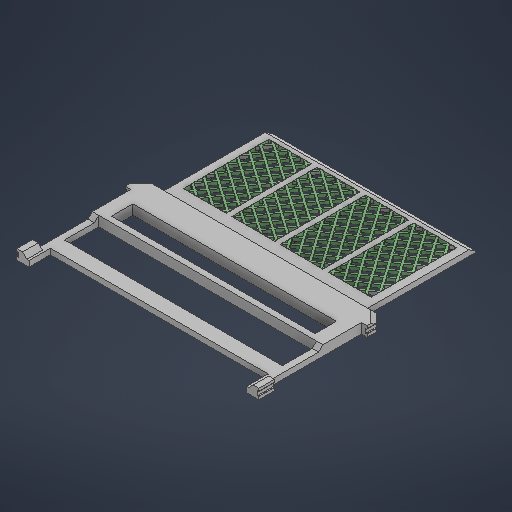
# Autodesk Inventor part: SACMI PH1500 FILLER BOX GRID-DRIVING
Saved by Autodesk Inventor 2025 (Build 290162000, 162)
## iProperties
Created: 2024-05-03
Part Number: SACMI PH1500 FILLER BOX GRID-DRIVING
Material: Generic
Document SubType Name: Modeling
Designer: zulet
Density: 1 g/cm^3
Appearance: Smooth - Medium Gray
Author: zulet
Autodesk Inventor part; units mm, degrees
(part 1 of 2)
ref_plane "YZ Plane" through (0, 0, 0) normal (1, 0, 0) x (0, 1, 0)
ref_plane "XZ Plane" through (0, 0, 0) normal (0, 1, 0) x (-1, 0, 0)
ref_plane "XY Plane" through (0, 0, 0) normal (0, 0, 1) x (1, 0, 0)
sketch "Sketch1" plane through (0, 0, 0) normal (0, 1, 0) x (-1, 0, 0)
  line L0 (-2029.8955, 1380.0763) -> (2005.9504, 1380.0763) construction
  line L1 (2005.9504, 1380.0763) -> (2005.9504, -2689.5627) construction
  line L2 (2005.9504, -2689.5627) -> (-2029.8955, -2689.5627) construction
  line L3 (-2029.8955, -2689.5627) -> (-2029.8955, 1380.0763) construction
  line L4 (810, 0) -> (765, 0)
  line L5 (715, -900) -> (780, -900)
  line L6 (780, -900) -> (850, -830)
  line L7 (850, -830) -> (850, -760)
  line L8 (850, -760) -> (810, -760)
  line L9 (810, -760) -> (810, 0)
  line L10 (715, -900) -> (715, -1610)
  line L11 (715, -1610) -> (0, -1610)
  line L12 (0, -1610) -> (0, -680)
  line L13 (0, -680) -> (715, -680)
  line L14 (765, -490) -> (0, -490)
  line L15 (0, -490) -> (0, -530)
  line L16 (0, -530) -> (715, -530)
  line L17 (715, -530) -> (715, -680)
  line L18 (765, -490) -> (765, -250)
  line L19 (765, -250) -> (0, -250)
  line L20 (0, -250) -> (0, -150)
  line L21 (0, -150) -> (765, -150)
  line L22 (765, -150) -> (765, 0)
  line L23 (810, 0) -> (850, 0)
  line L24 (850, 0) -> (850, -110)
  line L25 (850, -110) -> (810, -110)
  line L26 (810, -110) -> (810, 0)
  line L27 (0, 0) -> (0, -1610) construction
  line L28 (0, 0) -> (850, 0) construction
  line L29 (715, -900) -> (715, -680)
  line L30 (765, -490) -> (810, -490)
  line L31 (715, -900) -> (0, -900)
  point P0 (830, -110)
  point P1 (715, -605)
  point P2 (810, -110)
  point P3 (0, -900)
  dimension "d1" = 4035.8459
  dimension "d24" = 45
  dimension "d25" = 150
  dimension "d26" = 100
  dimension "d27" = 240
  dimension "d28" = 40
  dimension "d29" = 150
  dimension "d32" = 810
  dimension "d33" = 110
  dimension "d43" = 650
  dimension "d45" = 140
  dimension "d46" = 45
  dimension "d48" = 70
  dimension "d49" = 40
  dimension "d50" = 95
  dimension "d57" = 780
  constraints: 56 end point, 13 perpendicular, 7 horizontal, 6 collinear, 4 point on line, 3 vertical, 2 midpoint, 2 parallel, 2 other
  measures "d1" distance of L1.end L2.end
  measures "d24" distance between parallel lines of L22 L9
  measures "d25" distance between parallel lines of L4 L21
  measures "d26" distance between parallel lines of L19 L21
  measures "d27" distance between parallel lines of L14 L19
  measures "d28" distance between parallel lines of L16 L14
  measures "d29" distance between parallel lines of L13 L16
  measures "d32" distance between parallel lines of L27 L9
  measures "d33" distance of L23.end L24.end
  measures "d43" distance from line of point (830, -110) L8
  measures "d45" distance between parallel lines of L8 L5
  measures "d46" angle of L5 L6
  measures "d48" distance of L6.end L7.end
  measures "d49" distance between parallel lines of L9 L24
  measures "d50" distance from line of L9 point (715, -605)
  measures "d57" distance from line of L11 L6.end
extrude "Extrusion1" add sketch "Sketch1" along normal blind 70 contours L23 L24 L25 L9 | L9 L8 L7 L6 L5 L29 L17 L16 L15 L14 L30 | L31 L12 L13 L29
extrude "Extrusion3" add sketch "Sketch1" along normal blind 40 contours L9 L30 L18 L19 L20 L21 L22 L4 | L31 L12 L13 L29 | L10 L11 L12 L31
sketch "Sketch2" plane through (0, 40, 0) normal (0, 1, 0) x (1, 0, 0)
  line L0 (-660, 1580) -> (-360, 1580)
  line L1 (-360, 1580) -> (-360, 980)
  line L2 (-360, 980) -> (-660, 980)
  line L3 (-660, 980) -> (-660, 1580)
  line L4 (0, 1610) -> (-715, 1610) projected
  line L5 (-850, 830) -> (-850, 760) projected
  line L6 (-320, 980) -> (-20, 980)
  line L7 (-20, 980) -> (-20, 1580)
  line L8 (-20, 1580) -> (-320, 1580)
  line L9 (-320, 1580) -> (-320, 980)
  point P0 (0, 0)
  dimension "d58" = 300
  dimension "d59" = 600
  dimension "d60" = 30
  dimension "d61" = 190
  dimension "d62" = 300
  dimension "d63" = 600
  dimension "d64" = 40
  dimension "d65" = 30
  constraints: 16 end point, 4 parallel, 2 horizontal, 2 perpendicular
  measures "d58" distance of L1.end L2.end
  measures "d59" distance of L0.end L1.end
  measures "d60" distance between parallel lines of L4 L0
  measures "d61" distance between parallel lines of L3 L5
  measures "d62" distance of L8.end L7.end
  measures "d63" distance of L7.end L6.end
  measures "d64" distance between parallel lines of L1 L9
  measures "d65" distance between parallel lines of L4 L8
extrude "Extrusion4" cut sketch "Sketch2" against normal blind 40
sketch "Sketch3" plane through (0, 40, 0) normal (0, 1, 0) x (1, 0, 0)
  line L0 (317.5928, 1321.2787) -> (276.6352, 1349.9575)
  line L1 (276.6352, 1349.9575) -> (305.314, 1390.9151)
  line L2 (305.314, 1390.9151) -> (346.2716, 1362.2363)
  line L3 (346.2716, 1362.2363) -> (317.5928, 1321.2787)
  line L4 (-360, 980) -> (-660, 980) projected
  line L5 (264.3479, 1358.5611) -> (223.3903, 1387.24)
  line L6 (223.3903, 1387.24) -> (252.0691, 1428.1976)
  line L7 (252.0691, 1428.1976) -> (293.0267, 1399.5187)
  line L8 (293.0267, 1399.5187) -> (264.3479, 1358.5611)
  line L9 (211.103, 1395.8436) -> (170.1454, 1424.5224)
  line L10 (170.1454, 1424.5224) -> (198.8242, 1465.48)
  line L11 (198.8242, 1465.48) -> (239.7818, 1436.8012)
  line L12 (239.7818, 1436.8012) -> (211.103, 1395.8436)
  line L13 (157.8581, 1433.1261) -> (116.9005, 1461.8049)
  line L14 (116.9005, 1461.8049) -> (145.5794, 1502.7625)
  line L15 (145.5794, 1502.7625) -> (186.537, 1474.0837)
  line L16 (186.537, 1474.0837) -> (157.8581, 1433.1261)
  line L17 (104.6133, 1470.4085) -> (63.6557, 1499.0874)
  line L18 (63.6557, 1499.0874) -> (92.3345, 1540.045)
  line L19 (92.3345, 1540.045) -> (133.2921, 1511.3661)
  line L20 (133.2921, 1511.3661) -> (104.6133, 1470.4085)
  line L21 (51.3684, 1507.691) -> (10.4108, 1536.3698)
  line L22 (10.4108, 1536.3698) -> (39.0896, 1577.3274)
  line L23 (39.0896, 1577.3274) -> (80.0472, 1548.6486)
  line L24 (80.0472, 1548.6486) -> (51.3684, 1507.691)
  line L25 (-1.8765, 1544.9735) -> (-42.8341, 1573.6523)
  line L26 (-42.8341, 1573.6523) -> (-14.1553, 1614.6099)
  line L27 (-14.1553, 1614.6099) -> (26.8023, 1585.9311)
  line L28 (26.8023, 1585.9311) -> (-1.8765, 1544.9735)
  line L29 (-55.1214, 1582.2559) -> (-96.079, 1610.9348)
  line L30 (-96.079, 1610.9348) -> (-67.4002, 1651.8924)
  line L31 (-67.4002, 1651.8924) -> (-26.4426, 1623.2135)
  line L32 (-26.4426, 1623.2135) -> (-55.1214, 1582.2559)
  line L33 (-108.3663, 1619.5384) -> (-149.3239, 1648.2172)
  line L34 (-149.3239, 1648.2172) -> (-120.6451, 1689.1748)
  line L35 (-120.6451, 1689.1748) -> (-79.6874, 1660.496)
  line L36 (-79.6874, 1660.496) -> (-108.3663, 1619.5384)
  line L37 (-161.6112, 1656.8209) -> (-202.5688, 1685.4997)
  line L38 (-202.5688, 1685.4997) -> (-173.8899, 1726.4573)
  line L39 (-173.8899, 1726.4573) -> (-132.9323, 1697.7785)
  line L40 (-132.9323, 1697.7785) -> (-161.6112, 1656.8209)
  line L41 (-214.856, 1694.1033) -> (-255.8136, 1722.7822)
  line L42 (-255.8136, 1722.7822) -> (-227.1348, 1763.7398)
  line L43 (-227.1348, 1763.7398) -> (-186.1772, 1735.0609)
  line L44 (-186.1772, 1735.0609) -> (-214.856, 1694.1033)
  line L45 (-268.1009, 1731.3858) -> (-309.0585, 1760.0646)
  line L46 (-309.0585, 1760.0646) -> (-280.3797, 1801.0222)
  line L47 (-280.3797, 1801.0222) -> (-239.4221, 1772.3434)
  line L48 (-239.4221, 1772.3434) -> (-268.1009, 1731.3858)
  line L49 (-321.3458, 1768.6683) -> (-362.3034, 1797.3471)
  line L50 (-362.3034, 1797.3471) -> (-333.6246, 1838.3047)
  line L51 (-333.6246, 1838.3047) -> (-292.667, 1809.6259)
  line L52 (-292.667, 1809.6259) -> (-321.3458, 1768.6683)
  line L53 (-374.5907, 1805.9508) -> (-415.5483, 1834.6296)
  line L54 (-415.5483, 1834.6296) -> (-386.8695, 1875.5872)
  line L55 (-386.8695, 1875.5872) -> (-345.9119, 1846.9084)
  line L56 (-345.9119, 1846.9084) -> (-374.5907, 1805.9508)
  line L57 (-427.8356, 1843.2332) -> (-468.7932, 1871.912)
  line L58 (-468.7932, 1871.912) -> (-440.1143, 1912.8696)
  line L59 (-440.1143, 1912.8696) -> (-399.1567, 1884.1908)
  line L60 (-399.1567, 1884.1908) -> (-427.8356, 1843.2332)
  line L61 (280.3103, 1268.0338) -> (239.3527, 1296.7126)
  line L62 (239.3527, 1296.7126) -> (268.0315, 1337.6702)
  line L63 (268.0315, 1337.6702) -> (308.9891, 1308.9914)
  line L64 (308.9891, 1308.9914) -> (280.3103, 1268.0338)
  line L65 (227.0654, 1305.3162) -> (186.1078, 1333.9951)
  line L66 (186.1078, 1333.9951) -> (214.7867, 1374.9527)
  line L67 (214.7867, 1374.9527) -> (255.7443, 1346.2739)
  line L68 (255.7443, 1346.2739) -> (227.0654, 1305.3162)
  line L69 (173.8206, 1342.5987) -> (132.863, 1371.2775)
  line L70 (132.863, 1371.2775) -> (161.5418, 1412.2351)
  line L71 (161.5418, 1412.2351) -> (202.4994, 1383.5563)
  line L72 (202.4994, 1383.5563) -> (173.8206, 1342.5987)
  line L73 (120.5757, 1379.8812) -> (79.6181, 1408.56)
  line L74 (79.6181, 1408.56) -> (108.2969, 1449.5176)
  line L75 (108.2969, 1449.5176) -> (149.2545, 1420.8388)
  line L76 (149.2545, 1420.8388) -> (120.5757, 1379.8812)
  line L77 (67.3308, 1417.1637) -> (26.3732, 1445.8425)
  line L78 (26.3732, 1445.8425) -> (55.052, 1486.8001)
  line L79 (55.052, 1486.8001) -> (96.0096, 1458.1213)
  line L80 (96.0096, 1458.1213) -> (67.3308, 1417.1637)
  line L81 (14.0859, 1454.4461) -> (-26.8717, 1483.1249)
  line L82 (-26.8717, 1483.1249) -> (1.8071, 1524.0825)
  line L83 (1.8071, 1524.0825) -> (42.7647, 1495.4037)
  line L84 (42.7647, 1495.4037) -> (14.0859, 1454.4461)
  line L85 (-39.159, 1491.7286) -> (-80.1166, 1520.4074)
  line L86 (-80.1166, 1520.4074) -> (-51.4378, 1561.365)
  line L87 (-51.4378, 1561.365) -> (-10.4802, 1532.6862)
  line L88 (-10.4802, 1532.6862) -> (-39.159, 1491.7286)
  line L89 (-92.4039, 1529.0111) -> (-133.3615, 1557.6899)
  line L90 (-133.3615, 1557.6899) -> (-104.6826, 1598.6475)
  line L91 (-104.6826, 1598.6475) -> (-63.725, 1569.9687)
  line L92 (-63.725, 1569.9687) -> (-92.4039, 1529.0111)
  line L93 (-145.6487, 1566.2935) -> (-186.6063, 1594.9723)
  line L94 (-186.6063, 1594.9723) -> (-157.9275, 1635.93)
  line L95 (-157.9275, 1635.93) -> (-116.9699, 1607.2511)
  line L96 (-116.9699, 1607.2511) -> (-145.6487, 1566.2935)
  line L97 (-198.8936, 1603.576) -> (-239.8512, 1632.2548)
  line L98 (-239.8512, 1632.2548) -> (-211.1724, 1673.2124)
  line L99 (-211.1724, 1673.2124) -> (-170.2148, 1644.5336)
  line L100 (-170.2148, 1644.5336) -> (-198.8936, 1603.576)
  line L101 (-252.1385, 1640.8585) -> (-293.0961, 1669.5373)
  line L102 (-293.0961, 1669.5373) -> (-264.4173, 1710.4949)
  line L103 (-264.4173, 1710.4949) -> (-223.4597, 1681.8161)
  line L104 (-223.4597, 1681.8161) -> (-252.1385, 1640.8585)
  line L105 (-305.3834, 1678.1409) -> (-346.341, 1706.8198)
  line L106 (-346.341, 1706.8198) -> (-317.6622, 1747.7774)
  line L107 (-317.6622, 1747.7774) -> (-276.7046, 1719.0985)
  line L108 (-276.7046, 1719.0985) -> (-305.3834, 1678.1409)
  line L109 (-358.6283, 1715.4234) -> (-399.5859, 1744.1022)
  line L110 (-399.5859, 1744.1022) -> (-370.9071, 1785.0598)
  line L111 (-370.9071, 1785.0598) -> (-329.9494, 1756.381)
  line L112 (-329.9494, 1756.381) -> (-358.6283, 1715.4234)
  line L113 (-411.8732, 1752.7059) -> (-452.8308, 1781.3847)
  line L114 (-452.8308, 1781.3847) -> (-424.1519, 1822.3423)
  line L115 (-424.1519, 1822.3423) -> (-383.1943, 1793.6635)
  line L116 (-383.1943, 1793.6635) -> (-411.8732, 1752.7059)
  line L117 (-465.118, 1789.9883) -> (-506.0756, 1818.6672)
  line L118 (-506.0756, 1818.6672) -> (-477.3968, 1859.6248)
  line L119 (-477.3968, 1859.6248) -> (-436.4392, 1830.9459)
  line L120 (-436.4392, 1830.9459) -> (-465.118, 1789.9883)
  line L121 (243.0279, 1214.7889) -> (202.0703, 1243.4677)
  line L122 (202.0703, 1243.4677) -> (230.7491, 1284.4253)
  line L123 (230.7491, 1284.4253) -> (271.7067, 1255.7465)
  line L124 (271.7067, 1255.7465) -> (243.0279, 1214.7889)
  line L125 (189.783, 1252.0714) -> (148.8254, 1280.7502)
  line L126 (148.8254, 1280.7502) -> (177.5042, 1321.7078)
  line L127 (177.5042, 1321.7078) -> (218.4618, 1293.029)
  line L128 (218.4618, 1293.029) -> (189.783, 1252.0714)
  line L129 (136.5381, 1289.3538) -> (95.5805, 1318.0327)
  line L130 (95.5805, 1318.0327) -> (124.2593, 1358.9903)
  line L131 (124.2593, 1358.9903) -> (165.2169, 1330.3114)
  line L132 (165.2169, 1330.3114) -> (136.5381, 1289.3538)
  line L133 (83.2932, 1326.6363) -> (42.3356, 1355.3151)
  line L134 (42.3356, 1355.3151) -> (71.0144, 1396.2727)
  line L135 (71.0144, 1396.2727) -> (111.972, 1367.5939)
  line L136 (111.972, 1367.5939) -> (83.2932, 1326.6363)
  line L137 (30.0483, 1363.9188) -> (-10.9093, 1392.5976)
  line L138 (-10.9093, 1392.5976) -> (17.7695, 1433.5552)
  line L139 (17.7695, 1433.5552) -> (58.7271, 1404.8764)
  line L140 (58.7271, 1404.8764) -> (30.0483, 1363.9188)
  line L141 (-23.1966, 1401.2012) -> (-64.1542, 1429.8801)
  line L142 (-64.1542, 1429.8801) -> (-35.4753, 1470.8377)
  line L143 (-35.4753, 1470.8377) -> (5.4823, 1442.1588)
  line L144 (5.4823, 1442.1588) -> (-23.1966, 1401.2012)
  line L145 (-76.4414, 1438.4837) -> (-117.399, 1467.1625)
  line L146 (-117.399, 1467.1625) -> (-88.7202, 1508.1201)
  line L147 (-88.7202, 1508.1201) -> (-47.7626, 1479.4413)
  line L148 (-47.7626, 1479.4413) -> (-76.4414, 1438.4837)
  line L149 (-129.6863, 1475.7662) -> (-170.6439, 1504.445)
  line L150 (-170.6439, 1504.445) -> (-141.9651, 1545.4026)
  line L151 (-141.9651, 1545.4026) -> (-101.0075, 1516.7238)
  line L152 (-101.0075, 1516.7238) -> (-129.6863, 1475.7662)
  line L153 (-182.9312, 1513.0486) -> (-223.8888, 1541.7275)
  line L154 (-223.8888, 1541.7275) -> (-195.21, 1582.6851)
  line L155 (-195.21, 1582.6851) -> (-154.2524, 1554.0062)
  line L156 (-154.2524, 1554.0062) -> (-182.9312, 1513.0486)
  line L157 (-236.1761, 1550.3311) -> (-277.1337, 1579.0099)
  line L158 (-277.1337, 1579.0099) -> (-248.4549, 1619.9675)
  line L159 (-248.4549, 1619.9675) -> (-207.4973, 1591.2887)
  line L160 (-207.4973, 1591.2887) -> (-236.1761, 1550.3311)
  line L161 (-289.421, 1587.6136) -> (-330.3786, 1616.2924)
  line L162 (-330.3786, 1616.2924) -> (-301.6998, 1657.25)
  line L163 (-301.6998, 1657.25) -> (-260.7422, 1628.5712)
  line L164 (-260.7422, 1628.5712) -> (-289.421, 1587.6136)
  line L165 (-342.6659, 1624.896) -> (-383.6235, 1653.5749)
  line L166 (-383.6235, 1653.5749) -> (-354.9446, 1694.5325)
  line L167 (-354.9446, 1694.5325) -> (-313.987, 1665.8537)
  line L168 (-313.987, 1665.8537) -> (-342.6659, 1624.896)
  line L169 (-395.9107, 1662.1785) -> (-436.8683, 1690.8573)
  line L170 (-436.8683, 1690.8573) -> (-408.1895, 1731.8149)
  line L171 (-408.1895, 1731.8149) -> (-367.2319, 1703.1361)
  line L172 (-367.2319, 1703.1361) -> (-395.9107, 1662.1785)
  line L173 (-449.1556, 1699.461) -> (-490.1132, 1728.1398)
  line L174 (-490.1132, 1728.1398) -> (-461.4344, 1769.0974)
  line L175 (-461.4344, 1769.0974) -> (-420.4768, 1740.4186)
  line L176 (-420.4768, 1740.4186) -> (-449.1556, 1699.461)
  line L177 (-502.4005, 1736.7435) -> (-543.3581, 1765.4223)
  line L178 (-543.3581, 1765.4223) -> (-514.6793, 1806.3799)
  line L179 (-514.6793, 1806.3799) -> (-473.7217, 1777.7011)
  line L180 (-473.7217, 1777.7011) -> (-502.4005, 1736.7435)
  line L181 (205.7454, 1161.544) -> (164.7878, 1190.2228)
  line L182 (164.7878, 1190.2228) -> (193.4666, 1231.1804)
  line L183 (193.4666, 1231.1804) -> (234.4242, 1202.5016)
  line L184 (234.4242, 1202.5016) -> (205.7454, 1161.544)
  line L185 (152.5005, 1198.8265) -> (111.5429, 1227.5053)
  line L186 (111.5429, 1227.5053) -> (140.2217, 1268.4629)
  line L187 (140.2217, 1268.4629) -> (181.1793, 1239.7841)
  line L188 (181.1793, 1239.7841) -> (152.5005, 1198.8265)
  line L189 (99.2556, 1236.109) -> (58.298, 1264.7878)
  line L190 (58.298, 1264.7878) -> (86.9768, 1305.7454)
  line L191 (86.9768, 1305.7454) -> (127.9344, 1277.0666)
  line L192 (127.9344, 1277.0666) -> (99.2556, 1236.109)
  line L193 (46.0107, 1273.3914) -> (5.0531, 1302.0702)
  line L194 (5.0531, 1302.0702) -> (33.732, 1343.0278)
  line L195 (33.732, 1343.0278) -> (74.6896, 1314.349)
  line L196 (74.6896, 1314.349) -> (46.0107, 1273.3914)
  line L197 (-7.2341, 1310.6739) -> (-48.1917, 1339.3527)
  line L198 (-48.1917, 1339.3527) -> (-19.5129, 1380.3103)
  line L199 (-19.5129, 1380.3103) -> (21.4447, 1351.6315)
  line L200 (21.4447, 1351.6315) -> (-7.2341, 1310.6739)
  line L201 (-60.479, 1347.9564) -> (-101.4366, 1376.6352)
  line L202 (-101.4366, 1376.6352) -> (-72.7578, 1417.5928)
  line L203 (-72.7578, 1417.5928) -> (-31.8002, 1388.914)
  line L204 (-31.8002, 1388.914) -> (-60.479, 1347.9564)
  line L205 (-113.7239, 1385.2388) -> (-154.6815, 1413.9176)
  line L206 (-154.6815, 1413.9176) -> (-126.0027, 1454.8752)
  line L207 (-126.0027, 1454.8752) -> (-85.0451, 1426.1964)
  line L208 (-85.0451, 1426.1964) -> (-113.7239, 1385.2388)
  line L209 (-166.9688, 1422.5213) -> (-207.9264, 1451.2001)
  line L210 (-207.9264, 1451.2001) -> (-179.2476, 1492.1577)
  line L211 (-179.2476, 1492.1577) -> (-138.29, 1463.4789)
  line L212 (-138.29, 1463.4789) -> (-166.9688, 1422.5213)
  line L213 (-220.2137, 1459.8038) -> (-261.1713, 1488.4826)
  line L214 (-261.1713, 1488.4826) -> (-232.4925, 1529.4402)
  line L215 (-232.4925, 1529.4402) -> (-191.5349, 1500.7614)
  line L216 (-191.5349, 1500.7614) -> (-220.2137, 1459.8038)
  line L217 (-273.4586, 1497.0862) -> (-314.4162, 1525.7651)
  line L218 (-314.4162, 1525.7651) -> (-285.7373, 1566.7227)
  line L219 (-285.7373, 1566.7227) -> (-244.7797, 1538.0438)
  line L220 (-244.7797, 1538.0438) -> (-273.4586, 1497.0862)
  line L221 (-326.7034, 1534.3687) -> (-367.661, 1563.0475)
  line L222 (-367.661, 1563.0475) -> (-338.9822, 1604.0051)
  line L223 (-338.9822, 1604.0051) -> (-298.0246, 1575.3263)
  line L224 (-298.0246, 1575.3263) -> (-326.7034, 1534.3687)
  line L225 (-379.9483, 1571.6512) -> (-420.9059, 1600.33)
  line L226 (-420.9059, 1600.33) -> (-392.2271, 1641.2876)
  line L227 (-392.2271, 1641.2876) -> (-351.2695, 1612.6088)
  line L228 (-351.2695, 1612.6088) -> (-379.9483, 1571.6512)
  line L229 (-433.1932, 1608.9336) -> (-474.1508, 1637.6125)
  line L230 (-474.1508, 1637.6125) -> (-445.472, 1678.5701)
  line L231 (-445.472, 1678.5701) -> (-404.5144, 1649.8912)
  line L232 (-404.5144, 1649.8912) -> (-433.1932, 1608.9336)
  line L233 (-486.4381, 1646.2161) -> (-527.3957, 1674.8949)
  line L234 (-527.3957, 1674.8949) -> (-498.7169, 1715.8525)
  line L235 (-498.7169, 1715.8525) -> (-457.7593, 1687.1737)
  line L236 (-457.7593, 1687.1737) -> (-486.4381, 1646.2161)
  line L237 (-539.683, 1683.4986) -> (-580.6406, 1712.1774)
  line L238 (-580.6406, 1712.1774) -> (-551.9618, 1753.135)
  line L239 (-551.9618, 1753.135) -> (-511.0042, 1724.4562)
  line L240 (-511.0042, 1724.4562) -> (-539.683, 1683.4986)
  line L241 (168.4629, 1108.2991) -> (127.5053, 1136.978)
  line L242 (127.5053, 1136.978) -> (156.1841, 1177.9356)
  line L243 (156.1841, 1177.9356) -> (197.1417, 1149.2567)
  line L244 (197.1417, 1149.2567) -> (168.4629, 1108.2991)
  line L245 (115.218, 1145.5816) -> (74.2604, 1174.2604)
  line L246 (74.2604, 1174.2604) -> (102.9393, 1215.218)
  line L247 (102.9393, 1215.218) -> (143.8969, 1186.5392)
  line L248 (143.8969, 1186.5392) -> (115.218, 1145.5816)
  line L249 (61.9732, 1182.8641) -> (21.0156, 1211.5429)
  line L250 (21.0156, 1211.5429) -> (49.6944, 1252.5005)
  line L251 (49.6944, 1252.5005) -> (90.652, 1223.8217)
  line L252 (90.652, 1223.8217) -> (61.9732, 1182.8641)
  line L253 (8.7283, 1220.1465) -> (-32.2293, 1248.8254)
  line L254 (-32.2293, 1248.8254) -> (-3.5505, 1289.783)
  line L255 (-3.5505, 1289.783) -> (37.4071, 1261.1041)
  line L256 (37.4071, 1261.1041) -> (8.7283, 1220.1465)
  line L257 (-44.5166, 1257.429) -> (-85.4742, 1286.1078)
  line L258 (-85.4742, 1286.1078) -> (-56.7954, 1327.0654)
  line L259 (-56.7954, 1327.0654) -> (-15.8378, 1298.3866)
  line L260 (-15.8378, 1298.3866) -> (-44.5166, 1257.429)
  line L261 (-97.7615, 1294.7115) -> (-138.7191, 1323.3903)
  line L262 (-138.7191, 1323.3903) -> (-110.0403, 1364.3479)
  line L263 (-110.0403, 1364.3479) -> (-69.0827, 1335.6691)
  line L264 (-69.0827, 1335.6691) -> (-97.7615, 1294.7115)
  line L265 (-151.0064, 1331.9939) -> (-191.964, 1360.6728)
  line L266 (-191.964, 1360.6728) -> (-163.2852, 1401.6304)
  line L267 (-163.2852, 1401.6304) -> (-122.3276, 1372.9515)
  line L268 (-122.3276, 1372.9515) -> (-151.0064, 1331.9939)
  line L269 (-204.2513, 1369.2764) -> (-245.2089, 1397.9552)
  line L270 (-245.2089, 1397.9552) -> (-216.53, 1438.9128)
  line L271 (-216.53, 1438.9128) -> (-175.5724, 1410.234)
  line L272 (-175.5724, 1410.234) -> (-204.2513, 1369.2764)
  line L273 (-257.4961, 1406.5589) -> (-298.4537, 1435.2377)
  line L274 (-298.4537, 1435.2377) -> (-269.7749, 1476.1953)
  line L275 (-269.7749, 1476.1953) -> (-228.8173, 1447.5165)
  line L276 (-228.8173, 1447.5165) -> (-257.4961, 1406.5589)
  line L277 (-310.741, 1443.8413) -> (-351.6986, 1472.5202)
  line L278 (-351.6986, 1472.5202) -> (-323.0198, 1513.4778)
  line L279 (-323.0198, 1513.4778) -> (-282.0622, 1484.7989)
  line L280 (-282.0622, 1484.7989) -> (-310.741, 1443.8413)
  line L281 (-363.9859, 1481.1238) -> (-404.9435, 1509.8026)
  line L282 (-404.9435, 1509.8026) -> (-376.2647, 1550.7602)
  line L283 (-376.2647, 1550.7602) -> (-335.3071, 1522.0814)
  line L284 (-335.3071, 1522.0814) -> (-363.9859, 1481.1238)
  line L285 (-417.2308, 1518.4063) -> (-458.1884, 1547.0851)
  line L286 (-458.1884, 1547.0851) -> (-429.5096, 1588.0427)
  line L287 (-429.5096, 1588.0427) -> (-388.552, 1559.3639)
  line L288 (-388.552, 1559.3639) -> (-417.2308, 1518.4063)
  line L289 (-470.4757, 1555.6888) -> (-511.4333, 1584.3676)
  line L290 (-511.4333, 1584.3676) -> (-482.7545, 1625.3252)
  line L291 (-482.7545, 1625.3252) -> (-441.7969, 1596.6464)
  line L292 (-441.7969, 1596.6464) -> (-470.4757, 1555.6888)
  line L293 (-523.7206, 1592.9712) -> (-564.6782, 1621.65)
  line L294 (-564.6782, 1621.65) -> (-535.9993, 1662.6076)
  line L295 (-535.9993, 1662.6076) -> (-495.0417, 1633.9288)
  line L296 (-495.0417, 1633.9288) -> (-523.7206, 1592.9712)
  line L297 (-576.9654, 1630.2537) -> (-617.923, 1658.9325)
  line L298 (-617.923, 1658.9325) -> (-589.2442, 1699.8901)
  line L299 (-589.2442, 1699.8901) -> (-548.2866, 1671.2113)
  line L300 (-548.2866, 1671.2113) -> (-576.9654, 1630.2537)
  line L301 (131.1805, 1055.0542) -> (90.2228, 1083.7331)
  line L302 (90.2228, 1083.7331) -> (118.9017, 1124.6907)
  line L303 (118.9017, 1124.6907) -> (159.8593, 1096.0119)
  line L304 (159.8593, 1096.0119) -> (131.1805, 1055.0542)
  line L305 (77.9356, 1092.3367) -> (36.978, 1121.0155)
  line L306 (36.978, 1121.0155) -> (65.6568, 1161.9731)
  line L307 (65.6568, 1161.9731) -> (106.6144, 1133.2943)
  line L308 (106.6144, 1133.2943) -> (77.9356, 1092.3367)
  line L309 (24.6907, 1129.6192) -> (-16.2669, 1158.298)
  line L310 (-16.2669, 1158.298) -> (12.4119, 1199.2556)
  line L311 (12.4119, 1199.2556) -> (53.3695, 1170.5768)
  line L312 (53.3695, 1170.5768) -> (24.6907, 1129.6192)
  line L313 (-28.5542, 1166.9017) -> (-69.5118, 1195.5805)
  line L314 (-69.5118, 1195.5805) -> (-40.833, 1236.5381)
  line L315 (-40.833, 1236.5381) -> (0.1246, 1207.8593)
  line L316 (0.1246, 1207.8593) -> (-28.5542, 1166.9017)
  line L317 (-81.7991, 1204.1841) -> (-122.7567, 1232.8629)
  line L318 (-122.7567, 1232.8629) -> (-94.0779, 1273.8205)
  line L319 (-94.0779, 1273.8205) -> (-53.1203, 1245.1417)
  line L320 (-53.1203, 1245.1417) -> (-81.7991, 1204.1841)
  line L321 (-135.044, 1241.4666) -> (-176.0016, 1270.1454)
  line L322 (-176.0016, 1270.1454) -> (-147.3227, 1311.103)
  line L323 (-147.3227, 1311.103) -> (-106.3651, 1282.4242)
  line L324 (-106.3651, 1282.4242) -> (-135.044, 1241.4666)
  line L325 (-188.2888, 1278.7491) -> (-229.2464, 1307.4279)
  line L326 (-229.2464, 1307.4279) -> (-200.5676, 1348.3855)
  line L327 (-200.5676, 1348.3855) -> (-159.61, 1319.7067)
  line L328 (-159.61, 1319.7067) -> (-188.2888, 1278.7491)
  line L329 (-241.5337, 1316.0315) -> (-282.4913, 1344.7103)
  line L330 (-282.4913, 1344.7103) -> (-253.8125, 1385.668)
  line L331 (-253.8125, 1385.668) -> (-212.8549, 1356.9891)
  line L332 (-212.8549, 1356.9891) -> (-241.5337, 1316.0315)
  line L333 (-294.7786, 1353.314) -> (-335.7362, 1381.9928)
  line L334 (-335.7362, 1381.9928) -> (-307.0574, 1422.9504)
  line L335 (-307.0574, 1422.9504) -> (-266.0998, 1394.2716)
  line L336 (-266.0998, 1394.2716) -> (-294.7786, 1353.314)
  line L337 (-348.0235, 1390.5965) -> (-388.9811, 1419.2753)
  line L338 (-388.9811, 1419.2753) -> (-360.3023, 1460.2329)
  line L339 (-360.3023, 1460.2329) -> (-319.3447, 1431.5541)
  line L340 (-319.3447, 1431.5541) -> (-348.0235, 1390.5965)
  line L341 (-401.2684, 1427.8789) -> (-442.226, 1456.5578)
  line L342 (-442.226, 1456.5578) -> (-413.5472, 1497.5154)
  line L343 (-413.5472, 1497.5154) -> (-372.5896, 1468.8365)
  line L344 (-372.5896, 1468.8365) -> (-401.2684, 1427.8789)
  line L345 (-454.5133, 1465.1614) -> (-495.4709, 1493.8402)
  line L346 (-495.4709, 1493.8402) -> (-466.792, 1534.7978)
  line L347 (-466.792, 1534.7978) -> (-425.8344, 1506.119)
  line L348 (-425.8344, 1506.119) -> (-454.5133, 1465.1614)
  line L349 (-507.7581, 1502.4439) -> (-548.7157, 1531.1227)
  line L350 (-548.7157, 1531.1227) -> (-520.0369, 1572.0803)
  line L351 (-520.0369, 1572.0803) -> (-479.0793, 1543.4015)
  line L352 (-479.0793, 1543.4015) -> (-507.7581, 1502.4439)
  line L353 (-561.003, 1539.7263) -> (-601.9606, 1568.4052)
  line L354 (-601.9606, 1568.4052) -> (-573.2818, 1609.3628)
  line L355 (-573.2818, 1609.3628) -> (-532.3242, 1580.6839)
  line L356 (-532.3242, 1580.6839) -> (-561.003, 1539.7263)
  line L357 (-614.2479, 1577.0088) -> (-655.2055, 1605.6876)
  line L358 (-655.2055, 1605.6876) -> (-626.5267, 1646.6452)
  line L359 (-626.5267, 1646.6452) -> (-585.5691, 1617.9664)
  line L360 (-585.5691, 1617.9664) -> (-614.2479, 1577.0088)
  line L361 (93.898, 1001.8094) -> (52.9404, 1030.4882)
  line L362 (52.9404, 1030.4882) -> (81.6192, 1071.4458)
  line L363 (81.6192, 1071.4458) -> (122.5768, 1042.767)
  line L364 (122.5768, 1042.767) -> (93.898, 1001.8094)
  line L365 (40.6531, 1039.0918) -> (-0.3045, 1067.7707)
  line L366 (-0.3045, 1067.7707) -> (28.3743, 1108.7283)
  line L367 (28.3743, 1108.7283) -> (69.3319, 1080.0494)
  line L368 (69.3319, 1080.0494) -> (40.6531, 1039.0918)
  line L369 (-12.5918, 1076.3743) -> (-53.5494, 1105.0531)
  line L370 (-53.5494, 1105.0531) -> (-24.8706, 1146.0107)
  line L371 (-24.8706, 1146.0107) -> (16.087, 1117.3319)
  line L372 (16.087, 1117.3319) -> (-12.5918, 1076.3743)
  line L373 (-65.8367, 1113.6568) -> (-106.7943, 1142.3356)
  line L374 (-106.7943, 1142.3356) -> (-78.1154, 1183.2932)
  line L375 (-78.1154, 1183.2932) -> (-37.1578, 1154.6144)
  line L376 (-37.1578, 1154.6144) -> (-65.8367, 1113.6568)
  line L377 (-119.0815, 1150.9392) -> (-160.0392, 1179.6181)
  line L378 (-160.0392, 1179.6181) -> (-131.3603, 1220.5757)
  line L379 (-131.3603, 1220.5757) -> (-90.4027, 1191.8968)
  line L380 (-90.4027, 1191.8968) -> (-119.0815, 1150.9392)
  line L381 (-172.3264, 1188.2217) -> (-213.284, 1216.9005)
  line L382 (-213.284, 1216.9005) -> (-184.6052, 1257.8581)
  line L383 (-184.6052, 1257.8581) -> (-143.6476, 1229.1793)
  line L384 (-143.6476, 1229.1793) -> (-172.3264, 1188.2217)
  line L385 (-225.5713, 1225.5042) -> (-266.5289, 1254.183)
  line L386 (-266.5289, 1254.183) -> (-237.8501, 1295.1406)
  line L387 (-237.8501, 1295.1406) -> (-196.8925, 1266.4618)
  line L388 (-196.8925, 1266.4618) -> (-225.5713, 1225.5042)
  line L389 (-278.8162, 1262.7866) -> (-319.7738, 1291.4655)
  line L390 (-319.7738, 1291.4655) -> (-291.095, 1332.4231)
  line L391 (-291.095, 1332.4231) -> (-250.1374, 1303.7442)
  line L392 (-250.1374, 1303.7442) -> (-278.8162, 1262.7866)
  line L393 (-332.0611, 1300.0691) -> (-373.0187, 1328.7479)
  line L394 (-373.0187, 1328.7479) -> (-344.3399, 1369.7055)
  line L395 (-344.3399, 1369.7055) -> (-303.3823, 1341.0267)
  line L396 (-303.3823, 1341.0267) -> (-332.0611, 1300.0691)
  line L397 (-385.306, 1337.3516) -> (-426.2636, 1366.0304)
  line L398 (-426.2636, 1366.0304) -> (-397.5847, 1406.988)
  line L399 (-397.5847, 1406.988) -> (-356.6271, 1378.3092)
  line L400 (-356.6271, 1378.3092) -> (-385.306, 1337.3516)
  line L401 (-438.5508, 1374.6341) -> (-479.5084, 1403.3129)
  line L402 (-479.5084, 1403.3129) -> (-450.8296, 1444.2705)
  line L403 (-450.8296, 1444.2705) -> (-409.872, 1415.5917)
  line L404 (-409.872, 1415.5917) -> (-438.5508, 1374.6341)
  line L405 (-491.7957, 1411.9165) -> (-532.7533, 1440.5953)
  line L406 (-532.7533, 1440.5953) -> (-504.0745, 1481.5529)
  line L407 (-504.0745, 1481.5529) -> (-463.1169, 1452.8741)
  line L408 (-463.1169, 1452.8741) -> (-491.7957, 1411.9165)
  line L409 (-545.0406, 1449.199) -> (-585.9982, 1477.8778)
  line L410 (-585.9982, 1477.8778) -> (-557.3194, 1518.8354)
  line L411 (-557.3194, 1518.8354) -> (-516.3618, 1490.1566)
  line L412 (-516.3618, 1490.1566) -> (-545.0406, 1449.199)
  line L413 (-598.2855, 1486.4815) -> (-639.2431, 1515.1603)
  line L414 (-639.2431, 1515.1603) -> (-610.5643, 1556.1179)
  line L415 (-610.5643, 1556.1179) -> (-569.6067, 1527.4391)
  line L416 (-569.6067, 1527.4391) -> (-598.2855, 1486.4815)
  line L417 (-651.5304, 1523.7639) -> (-692.488, 1552.4427)
  line L418 (-692.488, 1552.4427) -> (-663.8092, 1593.4003)
  line L419 (-663.8092, 1593.4003) -> (-622.8516, 1564.7215)
  line L420 (-622.8516, 1564.7215) -> (-651.5304, 1523.7639)
  line L421 (56.6155, 948.5645) -> (15.6579, 977.2433)
  line L422 (15.6579, 977.2433) -> (44.3367, 1018.2009)
  line L423 (44.3367, 1018.2009) -> (85.2943, 989.5221)
  line L424 (85.2943, 989.5221) -> (56.6155, 948.5645)
  line L425 (3.3706, 985.847) -> (-37.587, 1014.5258)
  line L426 (-37.587, 1014.5258) -> (-8.9081, 1055.4834)
  line L427 (-8.9081, 1055.4834) -> (32.0495, 1026.8046)
  line L428 (32.0495, 1026.8046) -> (3.3706, 985.847)
  line L429 (-49.8743, 1023.1294) -> (-90.8319, 1051.8082)
  line L430 (-90.8319, 1051.8082) -> (-62.153, 1092.7658)
  line L431 (-62.153, 1092.7658) -> (-21.1954, 1064.087)
  line L432 (-21.1954, 1064.087) -> (-49.8743, 1023.1294)
  line L433 (-103.1191, 1060.4119) -> (-144.0767, 1089.0907)
  line L434 (-144.0767, 1089.0907) -> (-115.3979, 1130.0483)
  line L435 (-115.3979, 1130.0483) -> (-74.4403, 1101.3695)
  line L436 (-74.4403, 1101.3695) -> (-103.1191, 1060.4119)
  line L437 (-156.364, 1097.6944) -> (-197.3216, 1126.3732)
  line L438 (-197.3216, 1126.3732) -> (-168.6428, 1167.3308)
  line L439 (-168.6428, 1167.3308) -> (-127.6852, 1138.652)
  line L440 (-127.6852, 1138.652) -> (-156.364, 1097.6944)
  line L441 (-209.6089, 1134.9768) -> (-250.5665, 1163.6556)
  line L442 (-250.5665, 1163.6556) -> (-221.8877, 1204.6132)
  line L443 (-221.8877, 1204.6132) -> (-180.9301, 1175.9344)
  line L444 (-180.9301, 1175.9344) -> (-209.6089, 1134.9768)
  line L445 (-262.8538, 1172.2593) -> (-303.8114, 1200.9381)
  line L446 (-303.8114, 1200.9381) -> (-275.1326, 1241.8957)
  line L447 (-275.1326, 1241.8957) -> (-234.175, 1213.2169)
  line L448 (-234.175, 1213.2169) -> (-262.8538, 1172.2593)
  line L449 (-316.0987, 1209.5418) -> (-357.0563, 1238.2206)
  line L450 (-357.0563, 1238.2206) -> (-328.3774, 1279.1782)
  line L451 (-328.3774, 1279.1782) -> (-287.4198, 1250.4994)
  line L452 (-287.4198, 1250.4994) -> (-316.0987, 1209.5418)
  line L453 (-369.3435, 1246.8242) -> (-410.3012, 1275.5031)
  line L454 (-410.3012, 1275.5031) -> (-381.6223, 1316.4607)
  line L455 (-381.6223, 1316.4607) -> (-340.6647, 1287.7818)
  line L456 (-340.6647, 1287.7818) -> (-369.3435, 1246.8242)
  line L457 (-422.5884, 1284.1067) -> (-463.546, 1312.7855)
  line L458 (-463.546, 1312.7855) -> (-434.8672, 1353.7431)
  line L459 (-434.8672, 1353.7431) -> (-393.9096, 1325.0643)
  line L460 (-393.9096, 1325.0643) -> (-422.5884, 1284.1067)
  line L461 (-475.8333, 1321.3892) -> (-516.7909, 1350.068)
  line L462 (-516.7909, 1350.068) -> (-488.1121, 1391.0256)
  line L463 (-488.1121, 1391.0256) -> (-447.1545, 1362.3468)
  line L464 (-447.1545, 1362.3468) -> (-475.8333, 1321.3892)
  line L465 (-529.0782, 1358.6716) -> (-570.0358, 1387.3505)
  line L466 (-570.0358, 1387.3505) -> (-541.357, 1428.3081)
  line L467 (-541.357, 1428.3081) -> (-500.3994, 1399.6292)
  line L468 (-500.3994, 1399.6292) -> (-529.0782, 1358.6716)
  line L469 (-582.3231, 1395.9541) -> (-623.2807, 1424.6329)
  line L470 (-623.2807, 1424.6329) -> (-594.6019, 1465.5905)
  line L471 (-594.6019, 1465.5905) -> (-553.6443, 1436.9117)
  line L472 (-553.6443, 1436.9117) -> (-582.3231, 1395.9541)
  line L473 (-635.568, 1433.2366) -> (-676.5256, 1461.9154)
  line L474 (-676.5256, 1461.9154) -> (-647.8467, 1502.873)
  line L475 (-647.8467, 1502.873) -> (-606.8891, 1474.1942)
  line L476 (-606.8891, 1474.1942) -> (-635.568, 1433.2366)
  line L477 (-688.8128, 1470.519) -> (-729.7704, 1499.1979)
  line L478 (-729.7704, 1499.1979) -> (-701.0916, 1540.1555)
  line L479 (-701.0916, 1540.1555) -> (-660.134, 1511.4766)
  line L480 (-660.134, 1511.4766) -> (-688.8128, 1470.519)
  line L481 (19.333, 895.3196) -> (-21.6246, 923.9984)
  line L482 (-21.6246, 923.9984) -> (7.0543, 964.956)
  line L483 (7.0543, 964.956) -> (48.0119, 936.2772)
  line L484 (48.0119, 936.2772) -> (19.333, 895.3196)
  line L485 (-33.9118, 932.6021) -> (-74.8694, 961.2809)
  line L486 (-74.8694, 961.2809) -> (-46.1906, 1002.2385)
  line L487 (-46.1906, 1002.2385) -> (-5.233, 973.5597)
  line L488 (-5.233, 973.5597) -> (-33.9118, 932.6021)
  line L489 (-87.1567, 969.8845) -> (-128.1143, 998.5634)
  line L490 (-128.1143, 998.5634) -> (-99.4355, 1039.521)
  line L491 (-99.4355, 1039.521) -> (-58.4779, 1010.8421)
  line L492 (-58.4779, 1010.8421) -> (-87.1567, 969.8845)
  line L493 (-140.4016, 1007.167) -> (-181.3592, 1035.8458)
  line L494 (-181.3592, 1035.8458) -> (-152.6804, 1076.8034)
  line L495 (-152.6804, 1076.8034) -> (-111.7228, 1048.1246)
  line L496 (-111.7228, 1048.1246) -> (-140.4016, 1007.167)
  line L497 (-193.6465, 1044.4495) -> (-234.6041, 1073.1283)
  line L498 (-234.6041, 1073.1283) -> (-205.9253, 1114.0859)
  line L499 (-205.9253, 1114.0859) -> (-164.9677, 1085.4071)
  line L500 (-164.9677, 1085.4071) -> (-193.6465, 1044.4495)
  line L501 (-246.8914, 1081.7319) -> (-287.849, 1110.4108)
  line L502 (-287.849, 1110.4108) -> (-259.1701, 1151.3684)
  line L503 (-259.1701, 1151.3684) -> (-218.2125, 1122.6895)
  line L504 (-218.2125, 1122.6895) -> (-246.8914, 1081.7319)
  line L505 (-300.1363, 1119.0144) -> (-341.0939, 1147.6932)
  line L506 (-341.0939, 1147.6932) -> (-312.415, 1188.6508)
  line L507 (-312.415, 1188.6508) -> (-271.4574, 1159.972)
  line L508 (-271.4574, 1159.972) -> (-300.1363, 1119.0144)
  line L509 (-353.3811, 1156.2969) -> (-394.3387, 1184.9757)
  line L510 (-394.3387, 1184.9757) -> (-365.6599, 1225.9333)
  line L511 (-365.6599, 1225.9333) -> (-324.7023, 1197.2545)
  line L512 (-324.7023, 1197.2545) -> (-353.3811, 1156.2969)
  line L513 (-406.626, 1193.5793) -> (-447.5836, 1222.2582)
  line L514 (-447.5836, 1222.2582) -> (-418.9048, 1263.2158)
  line L515 (-418.9048, 1263.2158) -> (-377.9472, 1234.5369)
  line L516 (-377.9472, 1234.5369) -> (-406.626, 1193.5793)
  line L517 (-459.8709, 1230.8618) -> (-500.8285, 1259.5406)
  line L518 (-500.8285, 1259.5406) -> (-472.1497, 1300.4982)
  line L519 (-472.1497, 1300.4982) -> (-431.1921, 1271.8194)
  line L520 (-431.1921, 1271.8194) -> (-459.8709, 1230.8618)
  line L521 (-513.1158, 1268.1443) -> (-554.0734, 1296.8231)
  line L522 (-554.0734, 1296.8231) -> (-525.3946, 1337.7807)
  line L523 (-525.3946, 1337.7807) -> (-484.437, 1309.1019)
  line L524 (-484.437, 1309.1019) -> (-513.1158, 1268.1443)
  line L525 (-566.3607, 1305.4268) -> (-607.3183, 1334.1056)
  line L526 (-607.3183, 1334.1056) -> (-578.6394, 1375.0632)
  line L527 (-578.6394, 1375.0632) -> (-537.6818, 1346.3844)
  line L528 (-537.6818, 1346.3844) -> (-566.3607, 1305.4268)
  line L529 (-619.6055, 1342.7092) -> (-660.5632, 1371.388)
  line L530 (-660.5632, 1371.388) -> (-631.8843, 1412.3456)
  line L531 (-631.8843, 1412.3456) -> (-590.9267, 1383.6668)
  line L532 (-590.9267, 1383.6668) -> (-619.6055, 1342.7092)
  line L533 (-672.8504, 1379.9917) -> (-713.808, 1408.6705)
  line L534 (-713.808, 1408.6705) -> (-685.1292, 1449.6281)
  line L535 (-685.1292, 1449.6281) -> (-644.1716, 1420.9493)
  line L536 (-644.1716, 1420.9493) -> (-672.8504, 1379.9917)
  line L537 (-726.0953, 1417.2742) -> (-767.0529, 1445.953)
  line L538 (-767.0529, 1445.953) -> (-738.3741, 1486.9106)
  line L539 (-738.3741, 1486.9106) -> (-697.4165, 1458.2318)
  line L540 (-697.4165, 1458.2318) -> (-726.0953, 1417.2742)
  line L541 (-17.9494, 842.0747) -> (-58.907, 870.7535)
  line L542 (-58.907, 870.7535) -> (-30.2282, 911.7111)
  line L543 (-30.2282, 911.7111) -> (10.7294, 883.0323)
  line L544 (10.7294, 883.0323) -> (-17.9494, 842.0747)
  line L545 (-71.1943, 879.3572) -> (-112.1519, 908.036)
  line L546 (-112.1519, 908.036) -> (-83.4731, 948.9936)
  line L547 (-83.4731, 948.9936) -> (-42.5155, 920.3148)
  line L548 (-42.5155, 920.3148) -> (-71.1943, 879.3572)
  line L549 (-124.4392, 916.6397) -> (-165.3968, 945.3185)
  line L550 (-165.3968, 945.3185) -> (-136.718, 986.2761)
  line L551 (-136.718, 986.2761) -> (-95.7604, 957.5973)
  line L552 (-95.7604, 957.5973) -> (-124.4392, 916.6397)
  line L553 (-177.6841, 953.9221) -> (-218.6417, 982.6009)
  line L554 (-218.6417, 982.6009) -> (-189.9629, 1023.5585)
  line L555 (-189.9629, 1023.5585) -> (-149.0052, 994.8797)
  line L556 (-149.0052, 994.8797) -> (-177.6841, 953.9221)
  line L557 (-230.929, 991.2046) -> (-271.8866, 1019.8834)
  line L558 (-271.8866, 1019.8834) -> (-243.2077, 1060.841)
  line L559 (-243.2077, 1060.841) -> (-202.2501, 1032.1622)
  line L560 (-202.2501, 1032.1622) -> (-230.929, 991.2046)
  line L561 (-284.1738, 1028.4871) -> (-325.1314, 1057.1659)
  line L562 (-325.1314, 1057.1659) -> (-296.4526, 1098.1235)
  line L563 (-296.4526, 1098.1235) -> (-255.495, 1069.4447)
  line L564 (-255.495, 1069.4447) -> (-284.1738, 1028.4871)
  line L565 (-337.4187, 1065.7695) -> (-378.3763, 1094.4483)
  line L566 (-378.3763, 1094.4483) -> (-349.6975, 1135.406)
  line L567 (-349.6975, 1135.406) -> (-308.7399, 1106.7271)
  line L568 (-308.7399, 1106.7271) -> (-337.4187, 1065.7695)
  line L569 (-390.6636, 1103.052) -> (-431.6212, 1131.7308)
  line L570 (-431.6212, 1131.7308) -> (-402.9424, 1172.6884)
  line L571 (-402.9424, 1172.6884) -> (-361.9848, 1144.0096)
  line L572 (-361.9848, 1144.0096) -> (-390.6636, 1103.052)
  line L573 (-443.9085, 1140.3345) -> (-484.8661, 1169.0133)
  line L574 (-484.8661, 1169.0133) -> (-456.1873, 1209.9709)
  line L575 (-456.1873, 1209.9709) -> (-415.2297, 1181.2921)
  line L576 (-415.2297, 1181.2921) -> (-443.9085, 1140.3345)
  line L577 (-497.1534, 1177.6169) -> (-538.111, 1206.2958)
  line L578 (-538.111, 1206.2958) -> (-509.4321, 1247.2534)
  line L579 (-509.4321, 1247.2534) -> (-468.4745, 1218.5745)
  line L580 (-468.4745, 1218.5745) -> (-497.1534, 1177.6169)
  line L581 (-550.3983, 1214.8994) -> (-591.3559, 1243.5782)
  line L582 (-591.3559, 1243.5782) -> (-562.677, 1284.5358)
  line L583 (-562.677, 1284.5358) -> (-521.7194, 1255.857)
  line L584 (-521.7194, 1255.857) -> (-550.3983, 1214.8994)
  line L585 (-603.6431, 1252.1819) -> (-644.6007, 1280.8607)
  line L586 (-644.6007, 1280.8607) -> (-615.9219, 1321.8183)
  line L587 (-615.9219, 1321.8183) -> (-574.9643, 1293.1395)
  line L588 (-574.9643, 1293.1395) -> (-603.6431, 1252.1819)
  line L589 (-656.888, 1289.4643) -> (-697.8456, 1318.1432)
  line L590 (-697.8456, 1318.1432) -> (-669.1668, 1359.1008)
  line L591 (-669.1668, 1359.1008) -> (-628.2092, 1330.4219)
  line L592 (-628.2092, 1330.4219) -> (-656.888, 1289.4643)
  line L593 (-710.1329, 1326.7468) -> (-751.0905, 1355.4256)
  line L594 (-751.0905, 1355.4256) -> (-722.4117, 1396.3832)
  line L595 (-722.4117, 1396.3832) -> (-681.4541, 1367.7044)
  line L596 (-681.4541, 1367.7044) -> (-710.1329, 1326.7468)
  line L597 (-763.3778, 1364.0293) -> (-804.3354, 1392.7081)
  line L598 (-804.3354, 1392.7081) -> (-775.6566, 1433.6657)
  line L599 (-775.6566, 1433.6657) -> (-734.699, 1404.9869)
  line L600 (-734.699, 1404.9869) -> (-763.3778, 1364.0293)
  line L601 (-55.2319, 788.8298) -> (-96.1895, 817.5087)
  line L602 (-96.1895, 817.5087) -> (-67.5107, 858.4663)
  line L603 (-67.5107, 858.4663) -> (-26.5531, 829.7874)
  line L604 (-26.5531, 829.7874) -> (-55.2319, 788.8298)
  line L605 (-108.4768, 826.1123) -> (-149.4344, 854.7911)
  line L606 (-149.4344, 854.7911) -> (-120.7556, 895.7487)
  line L607 (-120.7556, 895.7487) -> (-79.798, 867.0699)
  line L608 (-79.798, 867.0699) -> (-108.4768, 826.1123)
  line L609 (-161.7217, 863.3948) -> (-202.6793, 892.0736)
  line L610 (-202.6793, 892.0736) -> (-174.0004, 933.0312)
  line L611 (-174.0004, 933.0312) -> (-133.0428, 904.3524)
  line L612 (-133.0428, 904.3524) -> (-161.7217, 863.3948)
  line L613 (-214.9665, 900.6772) -> (-255.9241, 929.3561)
  line L614 (-255.9241, 929.3561) -> (-227.2453, 970.3137)
  line L615 (-227.2453, 970.3137) -> (-186.2877, 941.6348)
  line L616 (-186.2877, 941.6348) -> (-214.9665, 900.6772)
  line L617 (-268.2114, 937.9597) -> (-309.169, 966.6385)
  line L618 (-309.169, 966.6385) -> (-280.4902, 1007.5961)
  line L619 (-280.4902, 1007.5961) -> (-239.5326, 978.9173)
  line L620 (-239.5326, 978.9173) -> (-268.2114, 937.9597)
  line L621 (-321.4563, 975.2422) -> (-362.4139, 1003.921)
  line L622 (-362.4139, 1003.921) -> (-333.7351, 1044.8786)
  line L623 (-333.7351, 1044.8786) -> (-292.7775, 1016.1998)
  line L624 (-292.7775, 1016.1998) -> (-321.4563, 975.2422)
  line L625 (-374.7012, 1012.5246) -> (-415.6588, 1041.2035)
  line L626 (-415.6588, 1041.2035) -> (-386.98, 1082.1611)
  line L627 (-386.98, 1082.1611) -> (-346.0224, 1053.4822)
  line L628 (-346.0224, 1053.4822) -> (-374.7012, 1012.5246)
  line L629 (-427.9461, 1049.8071) -> (-468.9037, 1078.4859)
  line L630 (-468.9037, 1078.4859) -> (-440.2249, 1119.4435)
  line L631 (-440.2249, 1119.4435) -> (-399.2672, 1090.7647)
  line L632 (-399.2672, 1090.7647) -> (-427.9461, 1049.8071)
  line L633 (-481.191, 1087.0896) -> (-522.1486, 1115.7684)
  line L634 (-522.1486, 1115.7684) -> (-493.4697, 1156.726)
  line L635 (-493.4697, 1156.726) -> (-452.5121, 1128.0472)
  line L636 (-452.5121, 1128.0472) -> (-481.191, 1087.0896)
  line L637 (-534.4358, 1124.3721) -> (-575.3934, 1153.0509)
  line L638 (-575.3934, 1153.0509) -> (-546.7146, 1194.0085)
  line L639 (-546.7146, 1194.0085) -> (-505.757, 1165.3297)
  line L640 (-505.757, 1165.3297) -> (-534.4358, 1124.3721)
  line L641 (-587.6807, 1161.6545) -> (-628.6383, 1190.3333)
  line L642 (-628.6383, 1190.3333) -> (-599.9595, 1231.2909)
  line L643 (-599.9595, 1231.2909) -> (-559.0019, 1202.6121)
  line L644 (-559.0019, 1202.6121) -> (-587.6807, 1161.6545)
  line L645 (-640.9256, 1198.937) -> (-681.8832, 1227.6158)
  line L646 (-681.8832, 1227.6158) -> (-653.2044, 1268.5734)
  line L647 (-653.2044, 1268.5734) -> (-612.2468, 1239.8946)
  line L648 (-612.2468, 1239.8946) -> (-640.9256, 1198.937)
  line L649 (-694.1705, 1236.2195) -> (-735.1281, 1264.8983)
  line L650 (-735.1281, 1264.8983) -> (-706.4493, 1305.8559)
  line L651 (-706.4493, 1305.8559) -> (-665.4917, 1277.1771)
  line L652 (-665.4917, 1277.1771) -> (-694.1705, 1236.2195)
  line L653 (-747.4154, 1273.5019) -> (-788.373, 1302.1807)
  line L654 (-788.373, 1302.1807) -> (-759.6941, 1343.1383)
  line L655 (-759.6941, 1343.1383) -> (-718.7365, 1314.4595)
  line L656 (-718.7365, 1314.4595) -> (-747.4154, 1273.5019)
  line L657 (-800.6603, 1310.7844) -> (-841.6179, 1339.4632)
  line L658 (-841.6179, 1339.4632) -> (-812.939, 1380.4208)
  line L659 (-812.939, 1380.4208) -> (-771.9814, 1351.742)
  line L660 (-771.9814, 1351.742) -> (-800.6603, 1310.7844)
  line L661 (-92.5144, 735.585) -> (-133.472, 764.2638)
  line L662 (-133.472, 764.2638) -> (-104.7931, 805.2214)
  line L663 (-104.7931, 805.2214) -> (-63.8355, 776.5426)
  line L664 (-63.8355, 776.5426) -> (-92.5144, 735.585)
  line L665 (-145.7592, 772.8674) -> (-186.7168, 801.5462)
  line L666 (-186.7168, 801.5462) -> (-158.038, 842.5038)
  line L667 (-158.038, 842.5038) -> (-117.0804, 813.825)
  line L668 (-117.0804, 813.825) -> (-145.7592, 772.8674)
  line L669 (-199.0041, 810.1499) -> (-239.9617, 838.8287)
  line L670 (-239.9617, 838.8287) -> (-211.2829, 879.7863)
  line L671 (-211.2829, 879.7863) -> (-170.3253, 851.1075)
  line L672 (-170.3253, 851.1075) -> (-199.0041, 810.1499)
  line L673 (-252.249, 847.4324) -> (-293.2066, 876.1112)
  line L674 (-293.2066, 876.1112) -> (-264.5278, 917.0688)
  line L675 (-264.5278, 917.0688) -> (-223.5702, 888.39)
  line L676 (-223.5702, 888.39) -> (-252.249, 847.4324)
  line L677 (-305.4939, 884.7148) -> (-346.4515, 913.3936)
  line L678 (-346.4515, 913.3936) -> (-317.7727, 954.3512)
  line L679 (-317.7727, 954.3512) -> (-276.8151, 925.6724)
  line L680 (-276.8151, 925.6724) -> (-305.4939, 884.7148)
  line L681 (-358.7388, 921.9973) -> (-399.6964, 950.6761)
  line L682 (-399.6964, 950.6761) -> (-371.0176, 991.6337)
  line L683 (-371.0176, 991.6337) -> (-330.06, 962.9549)
  line L684 (-330.06, 962.9549) -> (-358.7388, 921.9973)
  line L685 (-411.9837, 959.2798) -> (-452.9413, 987.9586)
  line L686 (-452.9413, 987.9586) -> (-424.2624, 1028.9162)
  line L687 (-424.2624, 1028.9162) -> (-383.3048, 1000.2374)
  line L688 (-383.3048, 1000.2374) -> (-411.9837, 959.2798)
  line L689 (-465.2285, 996.5622) -> (-506.1861, 1025.2411)
  line L690 (-506.1861, 1025.2411) -> (-477.5073, 1066.1987)
  line L691 (-477.5073, 1066.1987) -> (-436.5497, 1037.5198)
  line L692 (-436.5497, 1037.5198) -> (-465.2285, 996.5622)
  line L693 (-518.4734, 1033.8447) -> (-559.431, 1062.5235)
  line L694 (-559.431, 1062.5235) -> (-530.7522, 1103.4811)
  line L695 (-530.7522, 1103.4811) -> (-489.7946, 1074.8023)
  line L696 (-489.7946, 1074.8023) -> (-518.4734, 1033.8447)
  line L697 (-571.7183, 1071.1272) -> (-612.6759, 1099.806)
  line L698 (-612.6759, 1099.806) -> (-583.9971, 1140.7636)
  line L699 (-583.9971, 1140.7636) -> (-543.0395, 1112.0848)
  line L700 (-543.0395, 1112.0848) -> (-571.7183, 1071.1272)
  line L701 (-624.9632, 1108.4096) -> (-665.9208, 1137.0885)
  line L702 (-665.9208, 1137.0885) -> (-637.242, 1178.0461)
  line L703 (-637.242, 1178.0461) -> (-596.2844, 1149.3672)
  line L704 (-596.2844, 1149.3672) -> (-624.9632, 1108.4096)
  line L705 (-678.2081, 1145.6921) -> (-719.1657, 1174.3709)
  line L706 (-719.1657, 1174.3709) -> (-690.4869, 1215.3285)
  line L707 (-690.4869, 1215.3285) -> (-649.5292, 1186.6497)
  line L708 (-649.5292, 1186.6497) -> (-678.2081, 1145.6921)
  line L709 (-731.453, 1182.9746) -> (-772.4106, 1211.6534)
  line L710 (-772.4106, 1211.6534) -> (-743.7317, 1252.611)
  line L711 (-743.7317, 1252.611) -> (-702.7741, 1223.9322)
  line L712 (-702.7741, 1223.9322) -> (-731.453, 1182.9746)
  line L713 (-784.6978, 1220.257) -> (-825.6554, 1248.9359)
  line L714 (-825.6554, 1248.9359) -> (-796.9766, 1289.8935)
  line L715 (-796.9766, 1289.8935) -> (-756.019, 1261.2146)
  line L716 (-756.019, 1261.2146) -> (-784.6978, 1220.257)
  line L717 (-837.9427, 1257.5395) -> (-878.9003, 1286.2183)
  line L718 (-878.9003, 1286.2183) -> (-850.2215, 1327.1759)
  line L719 (-850.2215, 1327.1759) -> (-809.2639, 1298.4971)
  line L720 (-809.2639, 1298.4971) -> (-837.9427, 1257.5395)
  line L721 (-129.7968, 682.3401) -> (-170.7544, 711.0189)
  line L722 (-170.7544, 711.0189) -> (-142.0756, 751.9765)
  line L723 (-142.0756, 751.9765) -> (-101.118, 723.2977)
  line L724 (-101.118, 723.2977) -> (-129.7968, 682.3401)
  line L725 (-183.0417, 719.6225) -> (-223.9993, 748.3014)
  line L726 (-223.9993, 748.3014) -> (-195.3205, 789.259)
  line L727 (-195.3205, 789.259) -> (-154.3629, 760.5801)
  line L728 (-154.3629, 760.5801) -> (-183.0417, 719.6225)
  line L729 (-236.2866, 756.905) -> (-277.2442, 785.5838)
  line L730 (-277.2442, 785.5838) -> (-248.5654, 826.5414)
  line L731 (-248.5654, 826.5414) -> (-207.6078, 797.8626)
  line L732 (-207.6078, 797.8626) -> (-236.2866, 756.905)
  line L733 (-289.5315, 794.1875) -> (-330.4891, 822.8663)
  line L734 (-330.4891, 822.8663) -> (-301.8103, 863.8239)
  line L735 (-301.8103, 863.8239) -> (-260.8527, 835.1451)
  line L736 (-260.8527, 835.1451) -> (-289.5315, 794.1875)
  line L737 (-342.7764, 831.4699) -> (-383.734, 860.1488)
  line L738 (-383.734, 860.1488) -> (-355.0551, 901.1064)
  line L739 (-355.0551, 901.1064) -> (-314.0975, 872.4275)
  line L740 (-314.0975, 872.4275) -> (-342.7764, 831.4699)
  line L741 (-396.0212, 868.7524) -> (-436.9788, 897.4312)
  line L742 (-436.9788, 897.4312) -> (-408.3, 938.3888)
  line L743 (-408.3, 938.3888) -> (-367.3424, 909.71)
  line L744 (-367.3424, 909.71) -> (-396.0212, 868.7524)
  line L745 (-449.2661, 906.0349) -> (-490.2237, 934.7137)
  line L746 (-490.2237, 934.7137) -> (-461.5449, 975.6713)
  line L747 (-461.5449, 975.6713) -> (-420.5873, 946.9925)
  line L748 (-420.5873, 946.9925) -> (-449.2661, 906.0349)
  line L749 (-502.511, 943.3173) -> (-543.4686, 971.9962)
  line L750 (-543.4686, 971.9962) -> (-514.7898, 1012.9538)
  line L751 (-514.7898, 1012.9538) -> (-473.8322, 984.2749)
  line L752 (-473.8322, 984.2749) -> (-502.511, 943.3173)
  line L753 (-555.7559, 980.5998) -> (-596.7135, 1009.2786)
  line L754 (-596.7135, 1009.2786) -> (-568.0347, 1050.2362)
  line L755 (-568.0347, 1050.2362) -> (-527.0771, 1021.5574)
  line L756 (-527.0771, 1021.5574) -> (-555.7559, 980.5998)